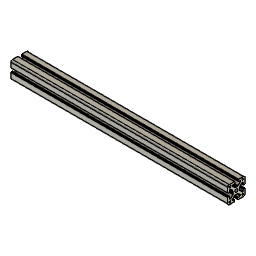
Profile 40x40 (Autodesk Fusion 360 design; units mm, degrees)
Autodesk Fusion 360 part; units mm, degrees
sketch "Sketch1" plane through (0, 0, 0) normal (1, 0, 0) x (0, 1, 0)
  line L0 (0, 0) -> (0, 40) construction
  line L1 (0, 0) -> (40, 0) construction
  line L2 (0, 7.6) -> (3.1, 7.6)
  arc A0 (3.1, 7.6) -> (3.8071, 7.8929) centre (3.1, 8.6) ccw
  line L3 (3.8071, 7.8929) -> (9.7071, 13.7929)
  arc A1 (9.7071, 13.7929) -> (9, 15.5) centre (9, 14.5) ccw
  line L4 (9, 15.5) -> (5.1, 15.5)
  arc A2 (4.1, 16.5) -> (5.1, 15.5) centre (5.1, 16.5) ccw
  line L5 (4.1, 16.5) -> (4.1, 19)
  arc A3 (5.1, 20) -> (4.1, 19) centre (5.1, 19) ccw
  line L6 (5.1, 20) -> (16.5, 20)
  arc A4 (20, 16.5) -> (16.5, 20) centre (16.5, 16.5) ccw
  line L7 (20, 16.5) -> (20, 4.1)
  arc A5 (19, 3.1) -> (20, 4.1) centre (19, 4.1) ccw
  line L8 (19, 3.1) -> (16.5, 3.1)
  arc A6 (15.5, 4.1) -> (16.5, 3.1) centre (16.5, 4.1) ccw
  line L9 (15.5, 4.1) -> (15.5, 9)
  line L10 (7.6, 0) -> (7.6, 3.1)
  arc A7 (15.5, 9) -> (13.7929, 9.7071) centre (14.5, 9) ccw
  line L11 (13.7929, 9.7071) -> (7.8929, 3.8071)
  arc A8 (7.8929, 3.8071) -> (7.6, 3.1) centre (8.6, 3.1) ccw
  arc A9 (3.4, 0) -> (0, 3.4) centre (0, 0) ccw
  line L12 (0, 0) -> (3.4, 0) construction
  line L13 (0, 0) -> (0, 3.4) construction
  line L14 (0, 7.6) -> (0, 3.4)
  line L15 (3.4, 0) -> (7.6, 0)
  line L16 (-7.6, 0) -> (-3.4, 0)
  arc A10 (-3.8071, 7.8929) -> (-3.1, 7.6) centre (-3.1, 8.6) ccw
  line L17 (-7.6, 0) -> (-7.6, 3.1)
  arc A11 (-7.6, 3.1) -> (-7.8929, 3.8071) centre (-8.6, 3.1) ccw
  line L18 (0, 7.6) -> (-3.1, 7.6)
  line L19 (0, 3.4) -> (0, 7.6)
  arc A12 (0, 3.4) -> (-3.4, 0) centre (0, 0) ccw
  arc A13 (-13.7929, 9.7071) -> (-15.5, 9) centre (-14.5, 9) ccw
  line L20 (-20, 5.1) -> (-20, 16.5)
  arc A14 (-16.5, 20) -> (-20, 16.5) centre (-16.5, 16.5) ccw
  arc A15 (-20, 5.1) -> (-19, 4.1) centre (-19, 5.1) ccw
  arc A16 (-16.5, 4.1) -> (-15.5, 5.1) centre (-16.5, 5.1) ccw
  arc A17 (-9, 15.5) -> (-9.7071, 13.7929) centre (-9, 14.5) ccw
  line L21 (-7.8929, 3.8071) -> (-13.7929, 9.7071)
  line L22 (-15.5, 9) -> (-15.5, 5.1)
  line L23 (-16.5, 4.1) -> (-19, 4.1)
  arc A18 (-3.1, 19) -> (-4.1, 20) centre (-4.1, 19) ccw
  line L24 (-16.5, 20) -> (-4.1, 20)
  line L25 (-4.1, 15.5) -> (-9, 15.5)
  line L26 (-3.1, 19) -> (-3.1, 16.5)
  arc A19 (-4.1, 15.5) -> (-3.1, 16.5) centre (-4.1, 16.5) ccw
  line L27 (-9.7071, 13.7929) -> (-3.8071, 7.8929)
  line L28 (0, -7.6) -> (0, -3.4)
  arc A20 (-7.8929, -3.8071) -> (-7.6, -3.1) centre (-8.6, -3.1) ccw
  line L29 (0, -7.6) -> (-3.1, -7.6)
  arc A21 (-3.1, -7.6) -> (-3.8071, -7.8929) centre (-3.1, -8.6) ccw
  line L30 (-7.6, 0) -> (-7.6, -3.1)
  line L31 (-3.4, 0) -> (-7.6, 0)
  arc A22 (-3.4, 0) -> (0, -3.4) centre (0, 0) ccw
  arc A23 (-9.7071, -13.7929) -> (-9, -15.5) centre (-9, -14.5) ccw
  line L32 (-5.1, -20) -> (-16.5, -20)
  arc A24 (-20, -16.5) -> (-16.5, -20) centre (-16.5, -16.5) ccw
  arc A25 (-5.1, -20) -> (-4.1, -19) centre (-5.1, -19) ccw
  arc A26 (-4.1, -16.5) -> (-5.1, -15.5) centre (-5.1, -16.5) ccw
  arc A27 (-15.5, -9) -> (-13.7929, -9.7071) centre (-14.5, -9) ccw
  line L33 (-3.8071, -7.8929) -> (-9.7071, -13.7929)
  line L34 (-9, -15.5) -> (-5.1, -15.5)
  line L35 (-4.1, -16.5) -> (-4.1, -19)
  arc A28 (-19, -3.1) -> (-20, -4.1) centre (-19, -4.1) ccw
  line L36 (-20, -16.5) -> (-20, -4.1)
  line L37 (-15.5, -4.1) -> (-15.5, -9)
  line L38 (-19, -3.1) -> (-16.5, -3.1)
  arc A29 (-15.5, -4.1) -> (-16.5, -3.1) centre (-16.5, -4.1) ccw
  line L39 (-13.7929, -9.7071) -> (-7.8929, -3.8071)
  line L40 (7.6, 0) -> (3.4, 0)
  arc A30 (3.8071, -7.8929) -> (3.1, -7.6) centre (3.1, -8.6) ccw
  line L41 (7.6, 0) -> (7.6, -3.1)
  arc A31 (7.6, -3.1) -> (7.8929, -3.8071) centre (8.6, -3.1) ccw
  line L42 (0, -7.6) -> (3.1, -7.6)
  line L43 (0, -3.4) -> (0, -7.6)
  arc A32 (0, -3.4) -> (3.4, 0) centre (0, 0) ccw
  arc A33 (13.7929, -9.7071) -> (15.5, -9) centre (14.5, -9) ccw
  line L44 (20, -5.1) -> (20, -16.5)
  arc A34 (16.5, -20) -> (20, -16.5) centre (16.5, -16.5) ccw
  arc A35 (20, -5.1) -> (19, -4.1) centre (19, -5.1) ccw
  arc A36 (16.5, -4.1) -> (15.5, -5.1) centre (16.5, -5.1) ccw
  arc A37 (9, -15.5) -> (9.7071, -13.7929) centre (9, -14.5) ccw
  line L45 (7.8929, -3.8071) -> (13.7929, -9.7071)
  line L46 (15.5, -9) -> (15.5, -5.1)
  line L47 (16.5, -4.1) -> (19, -4.1)
  arc A38 (3.1, -19) -> (4.1, -20) centre (4.1, -19) ccw
  line L48 (16.5, -20) -> (4.1, -20)
  line L49 (4.1, -15.5) -> (9, -15.5)
  line L50 (3.1, -19) -> (3.1, -16.5)
  arc A39 (4.1, -15.5) -> (3.1, -16.5) centre (4.1, -16.5) ccw
  line L51 (9.7071, -13.7929) -> (3.8071, -7.8929)
  circle A40 centre (15, 15) radius 2
  circle A41 centre (-15, 15) radius 2
  circle A42 centre (-15, -15) radius 2
  circle A43 centre (15, -15) radius 2
  dimension "d26" = 40
  dimension "d27" = 40
  dimension "d31" = 20
  dimension "d32" = 3.5
  dimension "d33" = 7.6
  dimension "d35" = 4.5
  dimension "d36" = 1
  dimension "d37" = 1
  dimension "d38" = 1
  dimension "d39" = 1
  dimension "d40" = 4.5
  dimension "d41" = 4.1
  dimension "d42" = 4.1
  dimension "d43" = 16.5
  dimension "d44" = 7.6
  dimension "d45" = 1
  dimension "d46" = 1
  dimension "d47" = 1
  dimension "d48" = 1
  dimension "d49" = 9
  dimension "d50" = 9
  dimension "d51" = 1
  dimension "d52" = 1
  dimension "d53" = 3.4
  dimension "d54" = 90
  dimension "d56" = 360
  dimension "d60" = 4
  dimension "d61" = 15
  dimension "d62" = 15
  constraint coincident L0.start L1.start
  constraint vertical L0
  constraint perpendicular L0 L1
  constraint coincident L0 L2.start
  constraint perpendicular L0 L2
  constraint tangent L2 A0
  constraint tangent A0 L3
  constraint tangent L3 A1
  constraint horizontal L4
  constraint tangent L4 A2
  constraint tangent A2 L5
  constraint perpendicular L4 L5
  constraint tangent L5 A3
  constraint tangent A3 L6
  constraint perpendicular L5 L6
  constraint tangent L6 A4
  constraint perpendicular L6 L7
  constraint tangent L7 A5
  constraint tangent A5 L8
  constraint perpendicular L7 L8
  constraint tangent L8 A6
  constraint tangent A6 L9
  constraint perpendicular L8 L9
  constraint coincident L1 L10.start
  constraint vertical L10
  constraint tangent L9 A7
  constraint tangent L11 A8
  constraint parallel L3 L11
  constraint equal L3 L11
  constraint equal L2 L10
  constraint parallel L0 L14
  measures "d26" distance of L0.start L0.end
  measures "d27" distance of L0.start L1.end
  measures "d31" distance of L0 A4.start
  measures "d32" radius of A4
  measures "d33" distance of L0.start L2.start
  measures "d35" distance of L4.end A3.start
  measures "d36" radius of A3
  measures "d37" radius of A2
  measures "d38" radius of A5
  measures "d39" radius of A6
  measures "d40" distance of L7.end A6.start
  measures "d41" distance of L1 L7.end
  measures "d42" distance of L0 L5.end
  measures "d43" distance of L0 A4.centre
  measures "d44" distance of L0 L10.start
  measures "d45" radius of A1
  measures "d46" radius of A7
  measures "d47" radius of A8
  measures "d48" radius of A0
  measures "d49" distance of L0 A1.centre
  measures "d50" distance of L1 A7.centre
  measures "d51" vertical distance of A1.end A1.centre
  measures "d52" horizontal distance of L10.end A8.centre
  measures "d53" radius of A9
  measures "d54" angle of L12 L13
  measures "d60" diameter of A40
  measures "d61" distance of L1 A40.centre
  measures "d62" distance of L0 A40.centre
extrude "Extrude2" add sketch "Sketch1" along normal blind 500 contours L2 A0 L3 A1 L4 A2 L5 A3 L6 A4 L7 A5 L8 A6 L9 L10 A7 L11 A8 A9 L14 L15 L19 L40 | L14 L16 A10 L17 A11 L18 L19 A12 A13 L20 A14 A15 A16 A17 L21 L22 L23 A18 L24 L25 L26 A19 L27 L31 | L15 L28 L40 A30 L41 A31 L42 L43 A32 A33 L44 A34 A35 A36 A37 L45 L46 L47 A38 L48 L49 L50 A39 L51 | L16 L28 A20 L29 A21 L30 L31 A22 A23 L32 A24 A25 A26 A27 L33 L34 L35 A28 L36 L37 L38 A29 L39 L43
equation "Length = 500 mm"
equation "d63 = Length"
named bodies: "Body"
